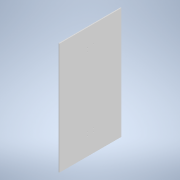
# Autodesk Inventor part: leftside
Saved by Autodesk Inventor 2020 (Build 240168000, 168)
## iProperties
Created: 2020-05-02
Part Number: leftside
Material: Generic
Document SubType Name: Modeling
Designer: galaxy
Density: 1 g/cm^3
Appearance: Default
Author: galaxy
Autodesk Inventor part; units mm, degrees
ref_plane "YZ Plane" through (0, 0, 0) normal (1, 0, 0) x (0, 1, 0)
ref_plane "XZ Plane" through (0, 0, 0) normal (0, 1, 0) x (-1, 0, 0)
ref_plane "XY Plane" through (0, 0, 0) normal (0, 0, 1) x (1, 0, 0)
sketch "Sketch1" plane through (0, 0, 0) normal (1, 0, 0) x (0, 1, 0)
  line L0 (180, 100) -> (-180, 100)
  line L1 (-180, 100) -> (-180, -100)
  line L2 (-180, -100) -> (180, -100)
  line L3 (180, -100) -> (180, 100)
  line L4 (180, 100) -> (-180, -100) construction
  line L5 (-180, 100) -> (180, -100) construction
  point P0 (0, 0)
  dimension "d0" = 360
  dimension "d1" = 200
  constraints: 12 end point, 2 midpoint, 2 parallel, 1 horizontal, 1 perpendicular
  measures "d0" distance of L2.end L1.end
  measures "d1" distance of L1.end L0.end
extrude "Extrusion1" add sketch "Sketch1" along normal blind 3
sketch "Sketch3" plane through (3, 0, 0) normal (1, 0, 0) x (0, 0, -1)
  circle A0 centre (-10.25, 123) radius 1.5
  circle A1 centre (-10.25, 111.5) radius 1.5
  circle A2 centre (10.25, 123) radius 1.5
  circle A3 centre (10.25, 111.5) radius 1.5
  line L0 (100, 180) -> (-100, 180) projected
  line L1 (100, -180) -> (100, 180) projected
  circle A4 centre (-10.25, -122.5) radius 1.5
  circle A5 centre (-10.25, -111) radius 1.5
  circle A6 centre (10.25, -122.5) radius 1.5
  circle A7 centre (10.25, -111) radius 1.5
  line L2 (-10.25, -122.5) -> (10.25, -122.5)
  line L3 (0, -122.5) -> (0, -180)
  line L4 (-100, -180) -> (100, -180) projected
  dimension "d11" = 3
  dimension "d12" = 3
  dimension "d13" = 3
  dimension "d14" = 3
  dimension "d15" = 11.5
  dimension "d16" = 11.5
  dimension "d21" = 20.5
  dimension "d24" = 57
  dimension "d25" = 57.5
  constraints: 8 centre point, 4 end point, 2 midpoint, 1 horizontal
  measures "d11" diameter of A0
  measures "d12" diameter of A1
  measures "d13" diameter of A2
  measures "d14" diameter of A3
  measures "d15" distance of A1.centre A0.centre
  measures "d16" distance between centres of A3 A2
  measures "d21" distance of A0.centre A2.centre
  measures "d24" distance from line of L0 A0.centre
  measures "d25" distance of L3.start L3.end
extrude "Extrusion3" cut sketch "Sketch3" against normal blind 25
body "Solid1"
